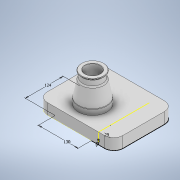
# Autodesk Inventor part: 77. Крышка верхняя
Saved by Autodesk Inventor 2021 (Build 250183000, 183)
## iProperties
Created: 2021-04-02
Part Number: 77. Крышка верхняя
Material: Типовые
Document SubType Name: Modeling
Designer: Данил
Density: 1 g/cm^3
Appearance: По умолчанию
Author: Данил
Autodesk Inventor part; units mm, degrees
ref_plane "YZ Plane" through (0, 0, 0) normal (1, 0, 0) x (0, 1, 0)
ref_plane "XZ Plane" through (0, 0, 0) normal (0, 1, 0) x (-1, 0, 0)
ref_plane "XY Plane" through (0, 0, 0) normal (0, 0, 1) x (1, 0, 0)
sketch "Эскиз5" plane through (0, 0, 0) normal (0, 1, 0) x (-1, 0, 0)
  line L0 (108, -126) -> (-139, -126)
  line L1 (-139, -126) -> (-139, 70)
  line L2 (-139, 70) -> (108, 70)
  line L3 (108, 70) -> (108, -126)
  point P0 (0, 0)
  point P1 (64, 58)
  point P2 (-104, 58)
  dimension "d19" = 64
  dimension "d20" = 58
  dimension "d21" = 203
  dimension "d22" = 12
  dimension "d23" = 184
  dimension "d24" = 168
  dimension "d25" = 212
  constraints: 8 end point, 2 parallel, 1 horizontal, 1 horizontal alignment, 1 perpendicular
  measures "d19" horizontal distance of point (64, 58) point (0, 0)
  measures "d20" vertical distance of point (64, 58) point (0, 0)
  measures "d21" distance from line of L1 point (64, 58)
  measures "d22" distance from line of L2 point (64, 58)
  measures "d23" distance from line of L0 point (64, 58)
  measures "d24" distance of point (-104, 58) point (64, 58)
  measures "d25" distance from line of L3 point (-104, 58)
extrude "Выдавливание2" add sketch "Эскиз5" along normal blind 36
sketch "Эскиз8" plane through (0, 0, 0) normal (0, 0, 1) x (1, 0, 0)
  line L0 (0, 0) -> (0, 133)
  line L1 (24.5, 98) -> (24.5, 132)
  line L2 (25.5, 133) -> (35.5, 133)
  line L3 (36.5, 132) -> (36.5, 130.4142)
  line L4 (36.2071, 129.7071) -> (32.5, 126)
  line L5 (32.5, 126) -> (32.5, 110)
  line L6 (32.5, 110) -> (36.5, 106)
  line L7 (36.5, 106) -> (46.3571, 55.2897)
  line L8 (46.5776, 54.1555) -> (46.5776, 93) construction
  line L9 (46.5776, 53) -> (46.5776, 36)
  line L10 (139, 36) -> (-108, 36) projected
  arc A0 (46.5776, 53) -> (46.3571, 55.2897) centre (34.5776, 53) ccw
  line L11 (24.5, 98) -> (27.9334, 98)
  line L12 (32.8415, 93.954) -> (40.3571, 55.2897)
  line L13 (40.5776, 53) -> (40.5776, 36)
  arc A1 (40.5776, 53) -> (40.3571, 55.2897) centre (28.5776, 53) ccw
  arc A2 (32.8415, 93.954) -> (27.9334, 98) centre (27.9334, 93) ccw
  line L14 (24.5, 132) -> (25.5, 133)
  arc A3 (36.5, 132) -> (35.5, 133) centre (35.5, 132) ccw
  arc A4 (36.2071, 129.7071) -> (36.5, 130.4142) centre (35.5, 130.4142) ccw
  point P0 (24.5, 133)
  point P1 (36.5, 133)
  dimension "d37" = 133
  dimension "d38" = 49
  dimension "d39" = 73
  dimension "d40" = 45
  dimension "d41" = 65
  dimension "d42" = 16
  dimension "d43" = 7
  dimension "d44" = 11
  dimension "d45" = 12
  dimension "d46" = 12
  dimension "d47" = 5
  dimension "d49" = 6
  dimension "d50" = 98
  dimension "d52" = 53
  dimension "d53" = 1
  dimension "d54" = 45
  dimension "d55" = 1
  constraints: 28 end point, 10 point on circle, 10 tangent, 9 point on line, 5 centre point, 5 perpendicular, 3 horizontal alignment, 3 vertical, 2 parallel, 1 coincident, 1 equal radius, 1 horizontal
  measures "d37" distance of L0.start L0.end
  measures "d38" diameter of L1 L0
  measures "d39" diameter of L3 L0
  measures "d40" angle of L3 L4
  measures "d41" diameter of L5 L0
  measures "d42" distance of L4.end L5.end
  measures "d43" vertical distance of point (36.5, 133) L4.end
  measures "d44" angle of L7 L8
  measures "d45" radius of A0
  measures "d46" radius of A1
  measures "d47" radius of A2
  measures "d49" distance between parallel lines of L13 L9
  measures "d50" distance from line of point (0, 0) L11
  measures "d52" vertical distance of point (0, 0) A0.centre
  measures "d53" distance of L1.end point (24.5, 133)
  measures "d54" angle of L1 L14
  measures "d55" radius of A3
revolve "Вращение1" add sketch "Эскиз8" angle 360 about axis through (0, 0, 0) along (0, 1, 0)
fillet "Сопряжение1" radius 30 4 edges at (-108, 18, 70) (-108, 18, -126) (139, 18, 70) (139, 18, -126)
sketch "Эскиз9" plane through (0, 0, 0) normal (0, 1, 0) x (-1, 0, 0)
  arc A0 (-139, -96) -> (-109, -126) centre (-109, -96) ccw construction
  line L0 (-139, 40) -> (-139, -96) construction
  arc A1 (-109, 70) -> (-139, 40) centre (-109, 40) ccw construction
  line L1 (78, 70) -> (-109, 70) construction
  arc A2 (108, 40) -> (78, 70) centre (78, 40) ccw construction
  line L2 (108, -96) -> (108, 40) construction
  arc A3 (78, -126) -> (108, -96) centre (78, -96) ccw construction
  line L3 (-109, -126) -> (78, -126) construction
  line L4 (-66, 70) -> (-109, 70)
  line L5 (-139, 40) -> (-139, -96)
  line L6 (-109, -126) -> (78, -126)
  arc A4 (78, -126) -> (108, -96) centre (78, -96) ccw
  arc A5 (-139, -96) -> (-109, -126) centre (-109, -96) ccw
  arc A6 (-109, 70) -> (-139, 40) centre (-109, 40) ccw
  line L7 (108, -96) -> (108, -66)
  point P0 (0, 0)
  point P1 (64, 58)
  dimension "d64" = 130
  dimension "d65" = 124
  constraints: 8 end point, 6 point on circle, 5 tangent, 3 centre point, 2 collinear, 2 point on line, 1 perpendicular
  measures "d64" horizontal distance of L4.start point (64, 58)
  measures "d65" vertical distance of L7.end point (64, 58)
ref_plane "РабПлоскость2" through (89, 0, 40) normal (1, 0, 0) x (0, 0, -1)
sketch "Эскиз10" plane through (89, 0, 40) normal (1, 0, 0) x (0, 0, -1)
  line L0 (0, 0) -> (-30, 0) projected
  line L1 (-30, 0) -> (-30, 8)
  line L2 (-30, 36) -> (-30, 0) projected
  arc A0 (-30, 8) -> (-25.258, 11.4146) centre (-30, 13) ccw
  line L3 (-30, 0) -> (-20.1156, 0)
  arc A1 (8.8844, 29) -> (-20.1156, 0) centre (8.8844, 0) ccw
  arc A2 (8.8844, 36) -> (-25.258, 11.4146) centre (8.8844, 0) ccw
  line L4 (0, 36) -> (136, 36) projected
  line L5 (8.8844, 36) -> (8.8844, 29)
  line L6 (-30, 36) -> (0, 36) projected
  point P0 (40, 0)
  dimension "d59" = 8
  dimension "d60" = 5
  dimension "d61" = 29
  constraints: 6 end point, 6 point on circle, 3 centre point, 3 point on line, 2 line through centre, 2 tangent, 1 coincident, 1 vertical
  measures "d59" distance of L0.end L1.end
  measures "d60" radius of A0
  measures "d61" radius of A1
